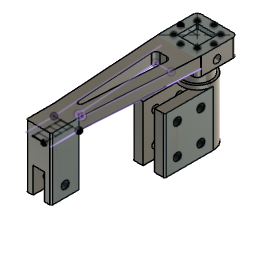
Fahnen_Halter_oben_v2 v20 (Autodesk Fusion 360 design; units mm, degrees)
Autodesk Fusion 360 part; units mm, degrees
note: some values were not read from the file. Set by a fixed rule: which sketch regions a step uses.
sketch "Skizze1" plane through (0, 0, 0) normal (0, 0, 1) x (1, 0, 0)
  line L0 (18.25, 16) -> (18.25, 51)
  line L1 (18.25, 51) -> (9.95, 51)
  line L2 (9.95, 51) -> (9.95, 16)
  line L3 (9.95, 16) -> (2.55, 16)
  line L4 (2.55, 16) -> (2.55, 51)
  line L5 (9.95, 51) -> (18.25, 51)
  line L6 (25.65, 51) -> (25.65, 16)
  line L7 (25.65, 16) -> (18.25, 16)
  arc A0 (25.65, 51) -> (2.55, 51) centre (14.1, 51) ccw
  dimension "d1" = 8.3
  dimension "d2" = 7.4
  dimension "d3" = 7.4
  dimension "d4" = 35
  dimension "d36" = 11.55
  constraint vertical L0
  constraint perpendicular L0 L1
  constraint perpendicular L1 L2
  constraint perpendicular L0 L3
  constraint perpendicular L1 L4
  constraint perpendicular L4 L5
  constraint perpendicular L1 L6
  constraint perpendicular L0 L7
  constraint tangent L6 A0
  constraint collinear L3 L7
  constraint midpoint L1 A0.centre
  measures "d1" distance of L0.end L1.end
  measures "d2" distance of L2.end L3.end
  measures "d3" distance of L0 L6
  measures "d4" distance of L1.end L2.end
  measures "d36" radius of A0
extrude "Extrusion1" add sketch "Skizze1" along normal blind 40 makes body 1
sketch "Skizze2" plane through (25.65, 0, 0) normal (1, 0, 0) x (0, 1, 0)
  line L0 (16, 0) -> (51, 0)
  line L1 (51, 0) -> (51, 40)
  line L2 (51, 40) -> (16, 40)
  line L3 (16, 40) -> (16, 0)
  circle A0 centre (25, 31) radius 2.6
  circle A1 centre (42, 31) radius 2.6
  circle A2 centre (25, 9) radius 2.6
  circle A3 centre (42, 9) radius 2.6
  dimension "d7" = 5.2
  dimension "d8" = 9
  dimension "d9" = 9
  dimension "d10" = 5.2
  dimension "d11" = 9
  dimension "d12" = 9
  dimension "d13" = 5.2
  dimension "d14" = 5.2
  dimension "d15" = 9
  dimension "d16" = 9
  dimension "d17" = 9
  dimension "d18" = 9
  measures "d7" diameter of A0
  measures "d8" distance of L3 A0.centre
  measures "d9" distance of L1 A1.centre
  measures "d10" diameter of A1
  measures "d11" distance of L2 A1.centre
  measures "d12" distance of L2 A0.centre
  measures "d13" diameter of A2
  measures "d14" diameter of A3
  measures "d15" distance of L3 A2.centre
  measures "d16" distance of L0 A2.centre
  measures "d17" distance of L0 A3.centre
  measures "d18" distance of L1 A3.centre
extrude "Extrusion2" cut sketch "Skizze2" against normal up to surface (23.1 mm away) contours A0 | A1 | A2 | A3 bodies 1
sketch "Skizze3" plane through (0, 0, 40) normal (0, 0, 1) x (-1, 0, 0)
  line L0 (-25.65, -16) -> (-25.65, -51)
  arc A0 (-25.65, -51) -> (-2.55, -51) centre (-14.1, -51) ccw
  line L1 (-2.55, -51) -> (-2.55, -16)
  line L2 (-2.55, -16) -> (-9.95, -16)
  line L3 (-9.95, -16) -> (-9.95, -51)
  line L4 (-9.95, -51) -> (-18.25, -51)
  line L5 (-18.25, -51) -> (-18.25, -16)
  line L6 (-18.25, -16) -> (-25.65, -16)
  circle A1 centre (-14.1, -51) radius 11.55
  constraint concentric A0 A1
  constraint tangent A0 A1
extrude "Extrusion6" add sketch "Skizze3" along normal blind 3 contours A0 L3 L4 L5 A1 | L3 L4 L5 A1 bodies 1
sketch "Skizze7" plane through (0, 0, 43) normal (0, 0, 1) x (-1, 0, 0)
  circle A0 centre (-14.1, -51) radius 11.55
  circle A1 centre (-14.1, -51) radius 9.85
  dimension "d39" = 19.7
  constraint concentric A0 A1
  measures "d39" diameter of A1
extrude "Extrusion7" add sketch "Skizze7" along normal blind 10.3 contours A1 bodies 1
sketch "Skizze5" plane through (0, 0, 53.3) normal (0, 0, 1) x (-1, 0, 0)
  circle A0 centre (-14.1, -51) radius 9.85
  line L0 (-21.065, -57.965) -> (-7.135, -57.965)
  line L1 (-7.135, -57.965) -> (-7.135, -44.035)
  line L2 (-7.135, -44.035) -> (-21.065, -44.035)
  line L3 (-21.065, -44.035) -> (-21.065, -57.965)
  line L4 (-21.065, -57.965) -> (-7.135, -44.035) construction
  line L5 (-7.135, -57.965) -> (-21.065, -44.035) construction
  line L6 (-6.885, -43.785) -> (-21.315, -43.785)
  line L7 (-21.315, -43.785) -> (-21.315, -58.215)
  line L8 (-21.315, -58.215) -> (-6.885, -58.215)
  line L9 (-6.885, -58.215) -> (-6.885, -43.785)
  line L10 (-28.565, -65.465) -> (0.365, -65.465)
  line L11 (0.365, -65.465) -> (0.365, -36.535)
  line L12 (0.365, -36.535) -> (-28.565, -36.535)
  line L13 (-28.565, -36.535) -> (-28.565, -65.465)
  point P0 (-14.1, -51)
  point P1 (-14.1, -51)
  dimension "d48" = 0.25
  dimension "d49" = 7.5
  constraint coincident P0 A0.centre
  constraint horizontal L0
  constraint perpendicular L0 L1
  constraint parallel L0 L2
  constraint parallel L1 L3
  constraint coincident L4 P1
  constraint coincident L5 P1
  constraint coincident P1 P0
  constraint equal L0 L3
  constraint coincident A0 L0.start
extrude "Extrusion8" add sketch "Skizze5" along normal blind 10 contours L0 L1 L2 L3 bodies 1
sketch "Skizze6" plane through (21.065, 0, 0) normal (1, 0, 0) x (0, 1, 0)
  line L0 (59.0964, 53.5) -> (59.0964, 63.5)
  line L1 (59.0964, 63.5) -> (42.9036, 63.5)
  line L2 (42.9036, 63.5) -> (42.9036, 53.5)
  circle A0 centre (50.7879, 58.5) radius 2.65
  line L3 (45.5676, 53.5) -> (56.4324, 53.5)
  line L4 (56.4324, 53.5) -> (59.0964, 53.5)
  line L5 (42.9036, 53.5) -> (45.5676, 53.5)
  line L6 (44.035, 53.3) -> (57.965, 53.3)
  line L7 (57.965, 53.3) -> (57.965, 63.3)
  line L8 (57.965, 63.3) -> (44.035, 63.3)
  line L9 (44.035, 63.3) -> (44.035, 53.3)
  dimension "d25" = 5.3
  dimension "d27" = 7.8842
  dimension "d28" = 7.8842
  dimension "d29" = 5
  measures "d25" diameter of A0
  measures "d27" distance of L2 A0.centre
  measures "d29" distance of L1 A0.centre
fillet "Abrundung1" radius 1 4 edges at (21.065, 57.965, 58.3) (21.065, 44.035, 58.3) (7.135, 44.035, 58.3) (7.135, 57.965, 58.3) on bodies 1
fillet "Abrundung2" radius 1 2 edges at (25.65, 16, 20) (2.55, 16, 20) on bodies 1
extrude "Extrusion9" add sketch "Skizze5" along normal blind 13 separate body contours A0 L9 | A0 L6 | A0 L8 | A0 L7 | L10 L11 L12 L13 makes body 2
fillet "Abrundung3" radius 0.6 4 edges at (21.315, 43.785, 59.8) (6.885, 43.785, 59.8) (6.885, 58.215, 59.8) (21.315, 58.215, 59.8) on bodies 2
extrude "Extrusion5" cut sketch "Skizze6" along normal blind -24 and the other way blind -12 contours A0 bodies 1 2
fillet "Abrundung4" radius 3 4 edges at (-0.365, 36.535, 59.8) (28.565, 36.535, 59.8) (28.565, 65.465, 59.8) (-0.365, 65.465, 59.8) on bodies 2
sketch "Skizze10" plane through (0, 0, 66.3) normal (0, 0, 1) x (-1, 0, 0)
  arc A0 (-2.635, -65.465) -> (0.365, -62.465) centre (-2.635, -62.465) ccw
  line L0 (0.365, -62.465) -> (0.365, -39.535)
  arc A1 (0.365, -39.535) -> (-2.635, -36.535) centre (-2.635, -39.535) ccw
  line L1 (-2.635, -36.535) -> (-25.565, -36.535)
  arc A2 (-25.565, -36.535) -> (-28.565, -39.535) centre (-25.565, -39.535) ccw
  line L2 (-28.565, -39.535) -> (-28.565, -62.465)
  arc A3 (-28.565, -62.465) -> (-25.565, -65.465) centre (-25.565, -62.465) ccw
  line L3 (-25.565, -65.465) -> (-2.635, -65.465)
  line L4 (-6.885, -44.385) -> (-6.885, -57.615)
  arc A4 (-7.485, -58.215) -> (-6.885, -57.615) centre (-7.485, -57.615) ccw
  line L5 (-7.485, -58.215) -> (-20.715, -58.215)
  arc A5 (-21.315, -57.615) -> (-20.715, -58.215) centre (-20.715, -57.615) ccw
  line L6 (-21.315, -57.615) -> (-21.315, -44.385)
  arc A6 (-20.715, -43.785) -> (-21.315, -44.385) centre (-20.715, -44.385) ccw
  line L7 (-20.715, -43.785) -> (-7.485, -43.785)
  arc A7 (-6.885, -44.385) -> (-7.485, -43.785) centre (-7.485, -44.385) ccw
  line L8 (-0.5137, -64.5863) -> (-27.6863, -37.4137) construction
  line L9 (-0.5137, -37.4137) -> (-27.6863, -64.5863) construction
  line L10 (-14.1, -51) -> (-2.1, -51) construction
  circle A8 centre (-2.1, -51) radius 1.05
  circle A9 centre (-5.6147, -42.5147) radius 1.05
  circle A10 centre (-14.1, -39) radius 1.05
  circle A11 centre (-22.5853, -42.5147) radius 1.05
  circle A12 centre (-26.1, -51) radius 1.05
  circle A13 centre (-22.5853, -59.4853) radius 1.05
  circle A14 centre (-14.1, -63) radius 1.05
  circle A15 centre (-5.6147, -59.4853) radius 1.05
  dimension "d81" = 12
  dimension "d82" = 2.1
  dimension "d84" = 360
  constraint midpoint A0 L8.start
  constraint midpoint A2 L8.end
  constraint midpoint A1 L9.start
  constraint midpoint A3 L9.end
  constraint midpoint L9 L10.start
  constraint perpendicular L4 L10
  constraint coincident L10.end A8.centre
  measures "d81" distance of L10.start L10.end
  measures "d82" diameter of A8
extrude "Extrusion14" cut sketch "Skizze10" against normal blind 10 contours A9 | A10 | A11 | A13 | A14 | A15 bodies 2
sketch "Skizze11" plane through (0, 0, 66.3) normal (0, 0, 1) x (-1, 0, 0)
  circle A0 centre (-5.6147, -59.4853) radius 1.05
  circle A1 centre (-14.1, -39) radius 1.05
  circle A2 centre (-14.1, -63) radius 1.05
  circle A3 centre (-5.6147, -42.5147) radius 1.05
  circle A4 centre (-22.5853, -42.5147) radius 1.05
  circle A5 centre (-22.5853, -59.4853) radius 1.05
  arc A6 (-2.635, -65.465) -> (0.365, -62.465) centre (-2.635, -62.465) ccw
  line L0 (0.365, -62.465) -> (0.365, -39.535)
  arc A7 (0.365, -39.535) -> (-2.635, -36.535) centre (-2.635, -39.535) ccw
  line L1 (-2.635, -36.535) -> (-25.565, -36.535)
  arc A8 (-25.565, -36.535) -> (-28.565, -39.535) centre (-25.565, -39.535) ccw
  line L2 (-28.565, -39.535) -> (-28.565, -62.465)
  arc A9 (-28.565, -62.465) -> (-25.565, -65.465) centre (-25.565, -62.465) ccw
  line L3 (-25.565, -65.465) -> (-2.635, -65.465)
  line L4 (-6.885, -44.385) -> (-6.885, -57.615)
  arc A10 (-7.485, -58.215) -> (-6.885, -57.615) centre (-7.485, -57.615) ccw
  line L5 (-7.485, -58.215) -> (-20.715, -58.215)
  arc A11 (-21.315, -57.615) -> (-20.715, -58.215) centre (-20.715, -57.615) ccw
  line L6 (-21.315, -57.615) -> (-21.315, -44.385)
  arc A12 (-20.715, -43.785) -> (-21.315, -44.385) centre (-20.715, -44.385) ccw
  line L7 (-20.715, -43.785) -> (-7.485, -43.785)
  arc A13 (-6.885, -44.385) -> (-7.485, -43.785) centre (-7.485, -44.385) ccw
  line L8 (0.365, -39.535) -> (0.365, 63.465) construction
  line L9 (-28.565, -39.535) -> (-28.565, 63.465) construction
  line L10 (0.365, 63.465) -> (-28.565, 63.465) construction
  line L11 (-5.1, 63.465) -> (-23.1, 63.465)
  line L12 (0.365, -39.535) -> (-5.1, 63.465) construction
  line L13 (-23.1, 63.465) -> (-28.565, -39.535) construction
  line L14 (-5.1, 63.465) -> (-5.1, 43.465)
  line L15 (0.365, -39.535) -> (-5.1, 43.465)
  line L16 (-23.1, 63.465) -> (-23.1, 43.465)
  line L17 (-23.1, 43.465) -> (-28.565, -39.535)
  line L18 (-12.4589, 33.465) -> (-8.5083, -26.535)
  line L19 (-15.7411, 33.465) -> (-19.6917, -26.535)
  line L20 (-12.4589, 33.465) -> (-15.7411, 33.465) construction
  line L21 (-8.5083, -26.535) -> (-19.6917, -26.535)
  arc A14 (-12.4589, 33.465) -> (-15.7411, 33.465) centre (-14.1, 33.465) ccw
  dimension "d87" = 18
  dimension "d90" = 100
  dimension "d95" = 20
  dimension "d96" = 20
  dimension "d120" = 8
  dimension "d121" = 8
  dimension "d122" = 30
  dimension "d123" = 10
  constraint coincident L0.end A7.start
  constraint tangent A7 L8
  constraint coincident A8.end L2.start
  constraint tangent A8 L9
  constraint equal L8 L9
  constraint coincident L10 L11.start
  constraint coincident L10 L11.end
  constraint midpoint L10 L11
  constraint perpendicular L10 L14
  constraint perpendicular L10 L16
  constraint parallel L15 L18
  constraint parallel L17 L19
  constraint horizontal L20
  constraint perpendicular L8 L21
  constraint midpoint L20 A14.centre
  measures "d87" distance of L11.start L11.end
  measures "d90" distance of L1 L10
  measures "d95" distance of L11.start L14.end
  measures "d96" distance of L11.end L16.end
  measures "d120" distance of L17 L19
  measures "d121" distance of L15 L18
  measures "d122" distance of L10 L20
  measures "d123" distance of L1 L21
extrude "Extrusion15" add sketch "Skizze11" against normal blind 8 contours A7 L1 A8 L11 L14 L15 L16 L17 bodies 2
sketch "Skizze12" plane through (0, 0, 58.3) normal (0, 0, -1) x (1, 0, 0)
  arc A0 (2.635, -36.535) -> (-0.3391, -39.1416) centre (2.635, -39.535) ccw
  line L0 (2.635, -36.535) -> (25.565, -36.535)
  arc A1 (28.5391, -39.1416) -> (25.565, -36.535) centre (25.565, -39.535) ccw
  line L1 (23.1, 63.465) -> (5.1, 63.465)
  line L2 (18.25, 63.465) -> (9.95, 63.465)
  line L3 (9.95, 63.465) -> (9.95, 43.465)
  line L4 (9.95, 43.465) -> (18.25, 43.465) construction
  line L5 (18.25, 43.465) -> (18.25, 63.465)
  line L6 (5.1, 63.465) -> (5.1, 43.465)
  line L7 (5.1, 43.465) -> (-0.3391, -39.1416)
  line L8 (28.5391, -39.1416) -> (23.1, 43.465)
  line L9 (23.1, 43.465) -> (23.1, 63.465)
  line L10 (5.1, 43.465) -> (23.1, 43.465)
  line L11 (9.95, 55.465) -> (18.25, 55.465)
  line L12 (18.25, 55.465) -> (18.25, 51.465)
  line L13 (18.25, 51.465) -> (9.95, 51.465)
  line L14 (9.95, 51.465) -> (9.95, 55.465)
  line L15 (9.95, 63.465) -> (18.25, 63.465)
  line L16 (18.25, 63.465) -> (18.25, 59.465)
  line L17 (18.25, 59.465) -> (9.95, 59.465)
  line L18 (9.95, 59.465) -> (9.95, 63.465)
  line L19 (9.95, 43.465) -> (18.25, 43.465)
  line L20 (18.25, 43.465) -> (18.25, 47.465)
  line L21 (18.25, 47.465) -> (9.95, 47.465)
  line L22 (9.95, 47.465) -> (9.95, 43.465)
  line L23 (8.5083, -26.535) -> (12.4589, 33.465)
  arc A2 (15.7411, 33.465) -> (12.4589, 33.465) centre (14.1, 33.465) ccw
  line L24 (15.7411, 33.465) -> (19.6917, -26.535)
  line L25 (19.6917, -26.535) -> (8.5083, -26.535)
  dimension "d92" = 8.3
  dimension "d110" = 4
  dimension "d112" = 4
  dimension "d113" = 4
  dimension "d115" = 4
  constraint horizontal L2
  constraint vertical L3
  constraint horizontal L4
  constraint vertical L5
  constraint coincident L1 L2.start
  constraint midpoint L1 L2
  constraint coincident L6.end L7.start
  constraint coincident L8.end L9.start
  constraint coincident L3.end L10
  constraint horizontal L11
  constraint vertical L12
  constraint horizontal L13
  constraint vertical L14
  constraint coincident L5 L12.end
  constraint coincident L3 L11.start
  constraint horizontal L15
  constraint vertical L16
  constraint horizontal L17
  constraint vertical L18
  constraint coincident L5 L16.end
  constraint horizontal L19
  constraint vertical L20
  constraint horizontal L21
  constraint vertical L22
  constraint coincident L5 L20.end
  constraint coincident L3 L4.start
  constraint collinear L10 L19
  measures "d92" distance of L3 L5
  measures "d110" distance of L2 L17
  measures "d112" distance of L11 L13
  measures "d113" distance of L11 L17
  measures "d115" distance of L19 L21
extrude "Extrusion17" add sketch "Skizze12" along normal blind 37 contours L1 L3 L6 L10 L14 L18 L22 | L1 L5 L9 L10 L12 L16 L20 bodies 2
sketch "Skizze13" plane through (23.1, 0, 0) normal (1, 0, 0) x (0, 1, 0)
  line L0 (-43.465, 66.3) -> (-63.465, 66.3)
  line L1 (-63.465, 66.3) -> (-63.465, 21.3)
  line L2 (-63.465, 21.3) -> (-43.465, 21.3)
  line L3 (-43.465, 21.3) -> (-43.465, 58.3)
  line L4 (-43.465, 58.3) -> (-43.465, 66.3)
  circle A0 centre (-53.465, 29.3) radius 2.6
  dimension "d99" = 5.2
  dimension "d100" = 8
  dimension "d102" = 10
  measures "d99" diameter of A0
  measures "d100" distance of L2 A0.centre
  measures "d102" distance of L1 A0.centre
extrude "Extrusion18" cut sketch "Skizze13" against normal up to surface (18 mm away) contours A0 bodies 2
fillet "Abrundung5" radius 1 2 edges at (23.1, -63.465, 43.8) (5.1, -63.465, 43.8) on bodies 2
extrude "Extrusion20" add sketch "Skizze12" along normal blind 18.3 contours L3 L5 L10 L19 L20 L21 L22 | L1 L2 L3 L5 L15 L16 L17 L18 | L3 L5 L11 L12 L13 L14 bodies 2
fillet "Abrundung6" radius 3 2 edges at (8.5083, 26.535, 62.3) (19.6917, 26.535, 62.3) on bodies 2
equation "d3 = d2"
equation "d10 = d7"
equation "d11 = d12"
equation "d14 = d7"
equation "d15 = d8"
equation "d16 = d12"
equation "d17 = d12"
equation "d18 = d9"
equation "d36 = d2 + d1 / 2"
equation "d96 = d95"
equation "d121 = d120"
named bodies: "Gelenk", "Arm"
